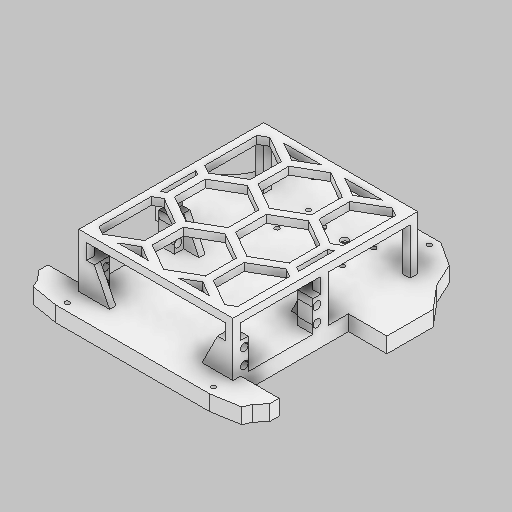
# Autodesk Inventor part: Base
Saved by Autodesk Inventor 2025 (Build 290162010, 162A)
## iProperties
Created: 2023-11-02
Part Number: Base
Material: Genérico
Document SubType Name: Modeling
Designer: juesr
Density: 1 g/cm^3
Appearance: Valor por defecto
Author: juesr
Autodesk Inventor part; units mm, degrees
ref_plane "YZ Plane" through (0, 0, 0) normal (1, 0, 0) x (0, 1, 0)
ref_plane "XZ Plane" through (0, 0, 0) normal (0, 1, 0) x (-1, 0, 0)
ref_plane "XY Plane" through (0, 0, 0) normal (0, 0, 1) x (1, 0, 0)
sketch "Boceto Base" plane through (0, 0, 0) normal (0, 1, 0) x (-1, 0, 0)
  line L0 (75, 80) -> (-75, 80)
  line L1 (-75, 80) -> (-75, -80)
  line L2 (-75, -80) -> (75, -80)
  line L3 (75, -80) -> (75, 80)
  point P0 (0, 0)
  point P1 (0, -80)
  point P2 (-75, 0)
  dimension "d0" = 160
  dimension "d7" = 75
  dimension "d8" = 80
  dimension "d9" = 150
  constraints: 8 end point, 2 midpoint, 2 parallel, 1 horizontal, 1 perpendicular
  measures "d0" distance from line of point (0, -80) L0
  measures "d7" distance from line of L1 point (0, 0)
  measures "d8" distance of point (0, -80) point (0, 0)
  measures "d9" distance between parallel lines of L1 L3
extrude "Base" add sketch "Boceto Base" along normal blind 10
sketch "Boceto Llantas" plane through (0, 10, 0) normal (0, 1, 0) x (1, 0, 0)
  line L0 (75, 80) -> (-75, 80) projected
  line L1 (-75, -80) -> (75, -80) projected
  line L2 (-75, 80) -> (-75, -80) projected
  line L3 (75, -80) -> (75, 80) projected
  line L4 (-75, 10) -> (-50, 10)
  line L5 (-50, 10) -> (-50, -60)
  line L6 (-50, -60) -> (-75, -60)
  line L7 (-75, -60) -> (-75, 10)
  line L8 (0, 80) -> (0, -80)
  line L9 (75, 80) -> (75, -80)
  line L10 (75, 10) -> (50, 10)
  line L11 (50, 10) -> (50, -60)
  line L12 (50, -60) -> (75, -60)
  line L13 (75, -60) -> (75, 10)
  point P0 (0, 0)
  point P1 (-62.5, -60)
  point P2 (-62.5, 10)
  point P3 (62.5, -60)
  point P4 (62.5, 10)
  point P5 (75, -60)
  point P6 (-75, -60)
  dimension "d4" = 70
  dimension "d5" = 70
  dimension "d6" = 20
  dimension "d10" = 25
  constraints: 20 end point, 6 symmetric about line, 4 midpoint, 2 parallel, 2 point on line, 1 horizontal, 1 perpendicular
  measures "d4" distance of point (-62.5, -60) point (-62.5, 10)
  measures "d5" distance between parallel lines of L0 L4
  measures "d6" distance between parallel lines of L1 L6
  measures "d10" distance between parallel lines of L5 L2
extrude "Llantas" cut sketch "Boceto Llantas" against normal blind 10 contours L3 L12 L11 L10 | L4 L5 L6 L2
sketch "Boceto Carroceria" plane through (0, 10, 0) normal (0, 1, 0) x (1, 0, 0)
  line L0 (-75, 80) -> (-75, 10) projected
  line L1 (-75, 40) -> (-62.4135, 55)
  line L2 (-62.4135, 55) -> (-55.4189, 70)
  line L3 (-55.4189, 70) -> (-40, 80)
  line L4 (75, 80) -> (-75, 80) projected
  line L5 (-75, 10) -> (-50, 10) projected
  line L6 (-75, 40) -> (-75, 80)
  line L7 (-40, 80) -> (-75, 80)
  line L8 (0, 80) -> (0, -80)
  line L9 (-75, -80) -> (75, -80) projected
  line L10 (-110.2671, 0) -> (114.8814, 0)
  line L11 (75, 80) -> (75, 10)
  line L12 (75, 40) -> (62.4135, 55)
  line L13 (62.4135, 55) -> (55.4189, 70)
  line L14 (55.4189, 70) -> (40, 80)
  line L15 (-75, 80) -> (75, 80)
  line L16 (75, 40) -> (75, 80)
  line L17 (40, 80) -> (75, 80)
  line L18 (110.2671, 0) -> (-114.8814, 0)
  line L19 (-75, -60) -> (-75, -80) projected
  line L20 (-75, -66) -> (-69.9654, -72)
  line L21 (-69.9654, -72) -> (-67.6339, -77)
  line L22 (-67.6339, -77) -> (-50, -80)
  line L23 (-50, -60) -> (-75, -60) projected
  line L24 (-75, -66) -> (-75, -80)
  line L25 (-50, -80) -> (-75, -80)
  line L26 (75, -80) -> (-75, -80)
  line L27 (75, -60) -> (75, -80)
  line L28 (75, -66) -> (69.9654, -72)
  line L29 (69.9654, -72) -> (67.6339, -77)
  line L30 (67.6339, -77) -> (50, -80)
  line L31 (75, -66) -> (75, -80)
  line L32 (50, -80) -> (75, -80)
  point P0 (0, 0)
  point P1 (50, -80)
  point P2 (40, 80)
  point P3 (-70.1592, -80)
  point P4 (70.1592, -80)
  point P5 (-67.9979, -80)
  point P6 (67.9979, -80)
  dimension "d13" = 30
  dimension "d14" = 50
  dimension "d15" = 65
  dimension "d16" = 40
  dimension "d17" = 15
  dimension "d18" = 15
  dimension "d19" = 6
  dimension "d20" = 50
  dimension "d21" = 50
  dimension "d22" = 65
  dimension "d23" = 6
  dimension "d24" = 5
  constraints: 54 end point, 16 symmetric about line, 8 point on line, 3 midpoint, 2 collinear, 1 horizontal, 1 perpendicular, 1 vertical
  measures "d13" distance of L0.end L1.start
  measures "d14" angle of L5 L1
  measures "d15" angle of L5 L2
  measures "d16" distance of L8.start L3.end
  measures "d17" vertical distance of L1.end L2.end
  measures "d18" vertical distance of L1.start L1.end
  measures "d19" distance of L19.start L20.start
  measures "d20" distance of L22.end point (0, -80)
  measures "d21" angle of L23 L20
  measures "d22" angle of L23 L21
  measures "d23" vertical distance of L20.start L20.end
  measures "d24" vertical distance of L20.end L21.end
extrude "Carroceria" cut sketch "Boceto Carroceria" against normal blind 10
sketch "Boceto Tornillos Chasis 1" plane through (0, 10, 0) normal (0, 1, 0) x (1, 0, 0)
  circle A0 centre (-37.5, 75) radius 1.5
  line L0 (40, 80) -> (-40, 80) projected
  line L1 (0, 82.2157) -> (0, 44.0996)
  circle A1 centre (37.5, 75) radius 1.5
  line L2 (-40, 80) -> (40, 80)
  circle A2 centre (-47.5, -75) radius 1.5
  line L3 (-50, -80) -> (50, -80) projected
  line L4 (0, -44.3891) -> (0, -85.4037)
  circle A3 centre (47.5, -75) radius 1.5
  point P0 (0, 0)
  point P1 (0, 80)
  point P2 (0, -80)
  point P3 (-65.5864, -80)
  point P4 (65.5864, -80)
  point P5 (-67.9979, -80)
  point P6 (67.9979, -80)
  dimension "d43" = 5
  dimension "d44" = 37.5
  dimension "d45" = 3
  dimension "d46" = 5
  dimension "d47" = 3
  dimension "d48" = 47.5
  constraints: 6 end point, 4 centre point, 4 symmetric about line, 2 midpoint, 2 vertical, 2 other
  measures "d43" distance from line of L0 A0.centre
  measures "d44" horizontal distance of point (0, 80) A0.centre
  measures "d45" diameter of A0
  measures "d46" distance from line of L3 A2.centre
  measures "d47" diameter of A2
  measures "d48" horizontal distance of point (0, -80) A2.centre
extrude "Tornillos Chasis 1" cut sketch "Boceto Tornillos Chasis 1" against normal blind 10
sketch "Boceto Tornillos Chasis 2" plane through (0, 0, 0) normal (0, -1, 0) x (1, 0, 0)
  circle A0 centre (-47.5, 75) radius 1.5 projected
  circle A1 centre (-47.5, 75) radius 2.5
  circle A2 centre (47.5, 75) radius 1.5 projected
  circle A3 centre (47.5, 75) radius 2.5
  circle A4 centre (-37.5, -75) radius 1.5 projected
  circle A5 centre (-37.5, -75) radius 2.5
  circle A6 centre (37.5, -75) radius 1.5 projected
  circle A7 centre (37.5, -75) radius 2.5
  point P0 (0, 0)
  dimension "d81" = 5
  dimension "d82" = 5
  dimension "d83" = 5
  dimension "d84" = 5
  constraints: 4 centre point, 4 coincident
  measures "d81" diameter of A1
  measures "d82" diameter of A3
  measures "d83" diameter of A5
  measures "d84" diameter of A7
extrude "Tornillos Chasis 2" cut sketch "Boceto Tornillos Chasis 2" against normal blind 2 contours A0 | A1 | A2 | A3 | A4 | A5 | A6 | A7
sketch "Boceto33" plane through (0, 0, 0) normal (0, -1, 0) x (1, 0, 0)
  circle A0 centre (7.5, -50) radius 1.5
  circle A1 centre (-7.5, -50) radius 1.5
  point P0 (0, 0)
  dimension "d287" = 3
  dimension "d288" = 3
  dimension "d289" = 50
  dimension "d290" = 50
  dimension "d291" = 7.5
  dimension "d292" = 7.5
  constraints: 2 centre point
  measures "d287" diameter of A0
  measures "d288" diameter of A1
  measures "d289" vertical distance of point (0, 0) A0.centre
  measures "d290" vertical distance of point (0, 0) A1.centre
  measures "d291" horizontal distance of point (0, 0) A1.centre
  measures "d292" horizontal distance of point (0, 0) A0.centre
extrude "Soporte Rueda 1" cut sketch "Boceto33" against normal blind 20
sketch "Boceto35" plane through (0, 10, 0) normal (0, 1, 0) x (1, 0, 0)
  circle A0 centre (-7.5, 50) radius 1.5 projected
  circle A1 centre (-7.5, 50) radius 2.5
  circle A2 centre (7.5, 50) radius 1.5 projected
  circle A3 centre (7.5, 50) radius 2.5
  point P0 (0, 0)
  dimension "d299" = 5
  dimension "d300" = 5
  constraints: 2 centre point, 2 coincident
  measures "d299" diameter of A1
  measures "d300" diameter of A3
extrude "Soporte Rueda 2" cut sketch "Boceto35" against normal blind 2 contours A0 | A1 | A2 | A3
sketch "Boceto27" plane through (0, 10, 0) normal (0, 1, 0) x (1, 0, 0)
  line L0 (50, -13) -> (40, -13)
  line L1 (40, -13) -> (40, -3)
  line L2 (40, -3) -> (50, -3)
  line L3 (50, -3) -> (50, -13)
  line L4 (50, -60) -> (50, 10) projected
  line L5 (50, -55) -> (40, -55)
  line L6 (40, -55) -> (40, -65)
  line L7 (40, -65) -> (50, -65)
  line L8 (50, -65) -> (50, -55)
  line L9 (75, -60) -> (50, -60) projected
  line L10 (0, -123.4453) -> (0, 138.5357)
  line L11 (-50, -13) -> (-40, -13)
  line L12 (-40, -13) -> (-40, -3)
  line L13 (-40, -3) -> (-50, -3)
  line L14 (-50, -3) -> (-50, -13)
  line L15 (-50, -60) -> (-50, 10)
  line L16 (-50, -55) -> (-40, -55)
  line L17 (-40, -55) -> (-40, -65)
  line L18 (-40, -65) -> (-50, -65)
  line L19 (-50, -65) -> (-50, -55)
  point P0 (0, 0)
  point P1 (45, -3)
  point P2 (45, -13)
  point P3 (45, -55)
  point P4 (45, -65)
  point P5 (-45, -3)
  point P6 (-45, -13)
  point P7 (-45, -55)
  point P8 (-45, -65)
  dimension "d244" = 10
  dimension "d245" = 10
  dimension "d247" = 10
  dimension "d248" = 10
  dimension "d249" = 5
  dimension "d250" = 42
  constraints: 36 end point, 14 symmetric about line, 4 midpoint, 4 parallel, 2 horizontal, 2 perpendicular, 2 point on line, 1 vertical
  measures "d244" distance of L0.start L0.end
  measures "d245" distance of point (45, -3) point (45, -13)
  measures "d247" distance of point (45, -55) point (45, -65)
  measures "d248" distance between parallel lines of L6 L4
  measures "d249" distance between parallel lines of L9 L5
  measures "d250" distance between parallel lines of L5 L0
extrude "Soporte Motor 1" add sketch "Boceto27" along normal blind 20
sketch "Boceto28" plane through (50, 0, 60) normal (1, 0, 0) x (0, 0, -1)
  circle A0 centre (2.5, 15) radius 2.5
  line L0 (5, 10) -> (5, 30) projected
  circle A1 centre (2.5, 25) radius 2.5
  circle A2 centre (49.5, 25) radius 2.5
  line L1 (47, 10) -> (47, 30) projected
  circle A3 centre (49.5, 15) radius 2.5
  line L2 (5, 10) -> (47, 10) projected
  point P0 (60, 0)
  dimension "d253" = 5
  dimension "d254" = 5
  dimension "d255" = 5
  dimension "d256" = 5
  dimension "d257" = 5
  dimension "d258" = 5
  dimension "d259" = 10
  dimension "d260" = 10
  constraints: 4 centre point, 4 tangent
  measures "d253" diameter of A1
  measures "d254" diameter of A0
  measures "d255" diameter of A3
  measures "d256" diameter of A2
  measures "d257" distance from line of L2 A3.centre
  measures "d258" distance from line of L2 A0.centre
  measures "d259" distance of A2.centre A3.centre
  measures "d260" distance of A0.centre A1.centre
extrude "Soporte Motor 2" cut sketch "Boceto28" against normal blind 100
sketch "Boceto29" plane through (0, 10, 0) normal (0, 1, 0) x (1, 0, 0)
  line L0 (40, -3) -> (30, -3)
  line L1 (30, -3) -> (30, -7)
  line L2 (30, -7) -> (40, -7)
  line L3 (40, -7) -> (40, -3)
  line L4 (40, -65) -> (40, -55) projected
  line L5 (40, -65) -> (30, -65)
  line L6 (30, -65) -> (30, -61)
  line L7 (30, -61) -> (40, -61)
  line L8 (40, -61) -> (40, -65)
  line L9 (0, 97.0479) -> (0, -97.0479)
  line L10 (-40, -3) -> (-30, -3)
  line L11 (-30, -3) -> (-30, -7)
  line L12 (-30, -7) -> (-40, -7)
  line L13 (-40, -7) -> (-40, -3)
  line L14 (-40, -65) -> (-40, -55)
  line L15 (-40, -65) -> (-30, -65)
  line L16 (-30, -65) -> (-30, -61)
  line L17 (-30, -61) -> (-40, -61)
  line L18 (-40, -61) -> (-40, -65)
  point P0 (0, 0)
  point P1 (35, -3)
  point P2 (35, -65)
  point P3 (35, -61)
  point P4 (40, -5)
  point P5 (30, -5)
  point P6 (40, -63)
  point P7 (30, -63)
  point P8 (-35, -3)
  point P9 (-35, -65)
  point P10 (-35, -61)
  point P11 (-40, -5)
  point P12 (-30, -5)
  point P13 (-40, -63)
  point P14 (-30, -63)
  dimension "d263" = 4
  dimension "d264" = 4
  dimension "d265" = 10
  dimension "d266" = 10
  constraints: 36 end point, 16 symmetric about line, 7 midpoint, 4 parallel, 2 horizontal, 2 perpendicular, 1 vertical
  measures "d263" distance from line of L2 point (35, -3)
  measures "d264" distance of point (35, -65) point (35, -61)
  measures "d265" distance of point (40, -5) point (30, -5)
  measures "d266" distance of point (40, -63) point (30, -63)
extrude "Soporte Motor 3" add sketch "Boceto29" along normal blind 20
sketch "Boceto30" plane through (50, 10, 3) normal (0, 0, -1) x (-1, 0, 0)
  line L0 (0, 20) -> (20, 20) projected
  line L1 (10, 20) -> (20, 0)
  line L2 (20, 0) -> (20, 20) projected
  line L3 (20, 0) -> (20, 20)
  line L4 (20, 20) -> (10, 20)
  line L5 (80, 0) -> (90, 0) projected
  line L6 (90, 20) -> (80, 0)
  line L7 (80, 0) -> (80, 20)
  line L8 (80, 20) -> (90, 20)
  line L9 (0, 0) -> (0, 20) projected
  line L10 (100, 0) -> (100, 20) projected
  line L11 (80, 20) -> (100, 20) projected
  point P0 (50, -10)
  point P1 (90, 20)
  dimension "d269" = 10
  dimension "d270" = 10
  constraints: 12 end point, 3 midpoint, 3 perpendicular, 2 point on line, 1 collinear
  measures "d269" distance from line of L9 point (10, 20)
  measures "d270" distance from line of L10 point (90, 20)
extrude "Soporte Motor 4" cut sketch "Boceto30" against normal blind 100
sketch "Boceto31" plane through (0, 10, 0) normal (0, 1, 0) x (1, 0, 0)
  circle A0 centre (-21.3, 35) radius 1.5
  line L0 (-95.6769, 0) -> (82.7696, 0)
  line L1 (0, 81.7869) -> (0, -11.5279)
  circle A1 centre (-21.3, 55.3) radius 1.5
  circle A2 centre (21.3, 35) radius 1.5
  circle A3 centre (21.3, 55.3) radius 1.5
  point P0 (0, 0)
  dimension "d273" = 3
  dimension "d274" = 35
  dimension "d275" = 21.3
  dimension "d276" = 21.3
  dimension "d277" = 3
  dimension "d278" = 20.3
  constraints: 4 centre point, 4 end point, 2 horizontal, 2 symmetric about line, 2 vertical, 2 other
  measures "d273" diameter of A0
  measures "d274" distance from line of L0 A0.centre
  measures "d275" distance from line of L1 A0.centre
  measures "d276" distance from line of L1 A1.centre
  measures "d277" diameter of A1
  measures "d278" distance of A0.centre A1.centre
extrude "Soporte ESP 1" cut sketch "Boceto31" against normal blind 20
sketch "Boceto32" plane through (0, 0, 0) normal (0, -1, 0) x (1, 0, 0)
  circle A0 centre (21.3, -55.3) radius 1.5 projected
  circle A1 centre (21.3, -55.3) radius 2.5
  circle A2 centre (22.5, -34.8477) radius 2.5
  circle A3 centre (-21.3, -55.3) radius 1.5 projected
  circle A4 centre (-21.3, -55.3) radius 2.5
  circle A5 centre (-22.5, -34.8477) radius 2.5
  point P0 (0, 0)
  dimension "d281" = 5
  dimension "d282" = 5
  dimension "d283" = 5
  dimension "d284" = 5
  constraints: 4 centre point, 2 coincident
  measures "d281" diameter of A1
  measures "d282" diameter of A2
  measures "d283" diameter of A4
  measures "d284" diameter of A5
extrude "Soporte ESP 2" cut sketch "Boceto32" against normal blind 2 contours A0 | A1 | A2 | A3 | A4 | A5
sketch "Boceto36" plane through (0, 10, 0) normal (0, 1, 0) x (1, 0, 0)
  line L0 (45, 50) -> (50, 50)
  line L1 (50, 50) -> (50, 55)
  line L2 (50, 55) -> (45, 55)
  line L3 (45, 55) -> (45, 50)
  line L4 (40, -65) -> (50, -65) projected
  line L5 (50, -65) -> (50, -55) projected
  line L6 (50, -60) -> (40, -60) projected
  line L7 (50, -65) -> (45, -65)
  line L8 (45, -65) -> (45, -60)
  line L9 (45, -60) -> (50, -60)
  line L10 (50, -60) -> (50, -65)
  line L11 (0, -102.1388) -> (0, 97.3853)
  line L12 (-45, 50) -> (-50, 50)
  line L13 (-50, 50) -> (-50, 55)
  line L14 (-50, 55) -> (-45, 55)
  line L15 (-45, 55) -> (-45, 50)
  line L16 (-40, -65) -> (-50, -65)
  line L17 (-50, -65) -> (-50, -55)
  line L18 (-50, -60) -> (-40, -60)
  line L19 (-50, -65) -> (-45, -65)
  line L20 (-45, -65) -> (-45, -60)
  line L21 (-45, -60) -> (-50, -60)
  line L22 (-50, -60) -> (-50, -65)
  line L23 (50, -8) -> (40, -8) projected
  line L24 (50, -3) -> (45, -3)
  line L25 (45, -3) -> (45, -8)
  line L26 (45, -8) -> (50, -8)
  line L27 (50, -8) -> (50, -3)
  line L28 (-50, -3) -> (-45, -3)
  line L29 (-45, -3) -> (-45, -8)
  line L30 (-45, -8) -> (-50, -8)
  line L31 (-50, -8) -> (-50, -3)
  point P0 (0, 0)
  point P1 (47.5, 50)
  point P2 (45, -65)
  point P3 (50, 52.5)
  point P4 (45, 52.5)
  point P5 (-47.5, 50)
  point P6 (-45, -65)
  point P7 (-50, 52.5)
  point P8 (-45, 52.5)
  dimension "d303" = 115
  dimension "d304" = 0
  dimension "d305" = 5
  dimension "d306" = 5
  constraints: 56 end point, 16 symmetric about line, 8 parallel, 6 midpoint, 4 horizontal, 4 perpendicular, 2 point on line, 1 vertical
  measures "d303" vertical distance of point (47.5, 50) point (45, -65)
  measures "d304" distance from line of L5 point (50, 52.5)
  measures "d305" distance between parallel lines of L2 L0
  measures "d306" distance of point (50, 52.5) point (45, 52.5)
extrude "Extrusión38" add sketch "Boceto36" along normal blind 30
sketch "Boceto37" plane through (0, 40, 0) normal (0, 1, 0) x (1, 0, 0)
  line L0 (-30, -65) -> (-50, -65) projected
  line L1 (45, 55) -> (50, 55) projected
  line L2 (-50, -65) -> (50, -65)
  line L3 (50, -65) -> (50, 55)
  line L4 (50, 55) -> (-50, 55)
  line L5 (-50, 55) -> (-50, -65)
  line L6 (-17.3205, -50) -> (-17.3205, -30)
  line L7 (-17.3205, -30) -> (0, -20)
  line L8 (0, -20) -> (17.3205, -30)
  line L9 (17.3205, -30) -> (17.3205, -50)
  line L10 (17.3205, -50) -> (0, -60)
  line L11 (0, -60) -> (-17.3205, -50)
  line L12 (45, 50) -> (45, 55) projected
  line L13 (-45, -60) -> (45, -60)
  line L14 (45, -60) -> (45, 50)
  line L15 (45, 50) -> (-45, 50)
  line L16 (-45, 50) -> (-45, -60)
  line L17 (-22.3205, -50) -> (-22.3205, -30)
  line L18 (-22.3205, -30) -> (-39.641, -20)
  line L19 (-39.641, -20) -> (-56.9615, -30)
  line L20 (-56.9615, -50) -> (-39.641, -60)
  line L21 (-39.641, -60) -> (-22.3205, -50)
  line L22 (56.9615, -30) -> (39.641, -20)
  line L23 (39.641, -20) -> (22.3205, -30)
  line L24 (22.3205, -30) -> (22.3205, -50)
  line L25 (22.3205, -50) -> (39.641, -60)
  line L26 (39.641, -60) -> (56.9615, -50)
  line L27 (19.8205, -54.3301) -> (37.141, -64.3301)
  line L28 (2.5, -64.3301) -> (19.8205, -54.3301)
  line L29 (-19.8205, -54.3301) -> (-2.5, -64.3301)
  line L30 (-37.141, -64.3301) -> (-19.8205, -54.3301)
  line L31 (19.8205, 14.3301) -> (2.5, 4.3301)
  line L32 (2.5, 4.3301) -> (2.5, -15.6699)
  line L33 (2.5, -15.6699) -> (19.8205, -25.6699)
  line L34 (19.8205, -25.6699) -> (37.141, -15.6699)
  line L35 (37.141, -15.6699) -> (37.141, 4.3301)
  line L36 (37.141, 4.3301) -> (19.8205, 14.3301)
  line L37 (-37.141, -15.6699) -> (-19.8205, -25.6699)
  line L38 (-19.8205, -25.6699) -> (-2.5, -15.6699)
  line L39 (-2.5, -15.6699) -> (-2.5, 4.3301)
  line L40 (-2.5, 4.3301) -> (-19.8205, 14.3301)
  line L41 (-19.8205, 14.3301) -> (-37.141, 4.3301)
  line L42 (-37.141, 4.3301) -> (-37.141, -15.6699)
  line L43 (-42.141, -15.6699) -> (-59.4615, -25.6699)
  line L44 (-42.141, 4.3301) -> (-42.141, -15.6699)
  line L45 (-59.4615, 14.3301) -> (-42.141, 4.3301)
  line L46 (59.4615, -25.6699) -> (42.141, -15.6699)
  line L47 (42.141, -15.6699) -> (42.141, 4.3301)
  line L48 (42.141, 4.3301) -> (59.4615, 14.3301)
  line L49 (-2.5, 52.9904) -> (-19.8205, 42.9904)
  line L50 (-19.8205, 42.9904) -> (-37.141, 52.9904)
  line L51 (17.3205, 18.6603) -> (0, 8.6603)
  line L52 (0, 8.6603) -> (-17.3205, 18.6603)
  line L53 (-17.3205, 18.6603) -> (-17.3205, 38.6603)
  line L54 (-17.3205, 38.6603) -> (0, 48.6603)
  line L55 (0, 48.6603) -> (17.3205, 38.6603)
  line L56 (17.3205, 38.6603) -> (17.3205, 18.6603)
  line L57 (-22.3205, 38.6603) -> (-39.641, 48.6603)
  line L58 (-39.641, 48.6603) -> (-56.9615, 38.6603)
  line L59 (-39.641, 8.6603) -> (-22.3205, 18.6603)
  line L60 (-22.3205, 18.6603) -> (-22.3205, 38.6603)
  line L61 (-56.9615, 18.6603) -> (-39.641, 8.6603)
  line L62 (56.9615, 38.6603) -> (39.641, 48.6603)
  line L63 (22.3205, 38.6603) -> (22.3205, 18.6603)
  line L64 (39.641, 48.6603) -> (22.3205, 38.6603)
  line L65 (39.641, 8.6603) -> (56.9615, 18.6603)
  line L66 (22.3205, 18.6603) -> (39.641, 8.6603)
  line L67 (37.141, 52.9904) -> (19.8205, 42.9904)
  line L68 (19.8205, 42.9904) -> (2.5, 52.9904)
  point P0 (0, 0)
  point P1 (0, -65)
  point P2 (0, -60)
  point P3 (-8.6603, -25)
  point P4 (-17.3205, 28.6603)
  point P5 (-45, -23.094)
  point P6 (-45, -56.906)
  point P7 (45, -23.094)
  point P8 (45, -56.906)
  point P9 (45, -17.3205)
  point P10 (45, 5.9808)
  point P11 (-45, -17.3205)
  point P12 (-45, 5.9808)
  point P13 (45, 11.7543)
  point P14 (45, 45.5662)
  point P15 (-10, -60)
  point P16 (-29.641, -60)
  point P17 (-45, 11.7543)
  point P18 (-45, 45.5662)
  point P19 (-31.9615, 50)
  point P20 (-7.6795, 50)
  point P21 (7.6795, 50)
  point P22 (31.9615, 50)
  point P23 (29.641, -60)
  point P24 (10, -60)
  dimension "d329" = 20
  dimension "d330" = 20
  dimension "d331" = 120
  dimension "d332" = 20
  dimension "d333" = 120
  dimension "d334" = 20
  dimension "d335" = 120
  dimension "d336" = 20
  dimension "d337" = 120
  dimension "d338" = 20
  dimension "d339" = 120
  dimension "d340" = 0
  dimension "d341" = 0
  constraints: 132 end point, 6 parallel, 4 midpoint, 2 horizontal, 2 perpendicular, 1 vertical
  measures "d329" distance of L6.start L6.end
  measures "d330" distance of L6.end L7.end
  measures "d331" angle of L6 L7
  measures "d332" distance of L7.end L8.end
  measures "d333" angle of L7 L8
  measures "d334" distance of L8.end L9.end
  measures "d335" angle of L8 L9
  measures "d336" distance of L9.end L10.end
  measures "d337" angle of L9 L10
  measures "d338" distance of L10.end L6.start
  measures "d339" angle of L10 L11
  measures "d340" horizontal distance of point (0, -65) L10.end
  measures "d341" distance of point (0, -60) L10.end
extrude "Extrusión39" add sketch "Boceto37" along normal blind 5 contours L0 L5 L20 L16 L13 L14 L26 L3 L2 | L5 L19 L16 L20 | L26 L14 L22 L3 | L5 L43 L16 L19 | L20 L13 L16 | L22 L14 L46 L3 | L14 L13 L26 | L5 L45 L16 L43 | L16 L43 L44 L45 L61 L59 L60 L57 L58 L15 L50 L49 L68 L67 L14 L62 L64 L63 L66 L65 L48 L47 L46 L22 L23 L24 L25 L13 L27 L28 L29 L30 L21 L17 L18 L19 | L46 L14 L48 L3 | L5 L61 L16 L45 | L48 L14 L65 L3 | L5 L58 L16 L61 | L65 L14 L62 L3 | L5 L4 L12 L15 L16 L58 | L62 L14 L12 L1 L3
